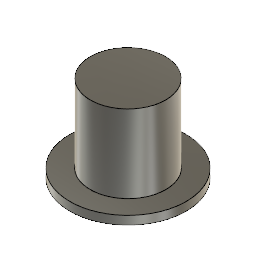
RetroconsoleButtoncap (Autodesk Fusion 360 design; units mm, degrees)
Autodesk Fusion 360 part; units mm, degrees
sketch "Sketch1" plane through (0, 0, 0) normal (0, 0, 1) x (1, 0, 0)
  circle A0 centre (0, 0) radius 4.375
  circle A1 centre (0, 0) radius 6.75
  dimension "d1" = 8.75
  dimension "d2" = 13.5
  constraint coincident A0.centre A1.centre
  measures "d1" diameter of A0
  measures "d2" diameter of A1
extrude "Extrude2" add sketch "Sketch1" along normal blind 7 contours A0 makes body 1
extrude "Extrude1" add sketch "Sketch1" along normal blind 1.5 separate body makes body 2
sketch "Sketch2" plane through (0, 0, 0) normal (0, 0, 1) x (1, 0, 0)
  circle A0 centre (0, 0) radius 3.525
  dimension "d7" = 7.05
  constraint coincident A0.centre origin
  measures "d7" diameter of A0
extrude "Extrude3" add 1 faces at (5.9169, -0.5527, 1.5) along direction (0, 0, 1) blind 0.5 on bodies 2 bodies 2 1
extrude "Extrude4" cut sketch "Sketch2" along normal blind 2 bodies 2
move_body "Move1" bodies 2 to x (1, 0, 0) y (0, -1, 0) z (0, 0, -1) at (0, 0, 0)
move_body "Move2" bodies 2 to x (1, 0, 0) y (0, -1, 0) z (0, 0, -1) at (0, -12, -14)
extrude "Extrude5" cut 1 faces at (5.9169, -12.5527, -12) along direction (0, 0, -1) blind 1 on bodies 2 bodies 2
extrude "Extrude6" add 1 faces at (-1.6096, -11.0197, -7) along direction (0, 0, 1) blind 3 on bodies 2 bodies 2
extrude "Extrude7" add 1 faces at (5.9169, -12.5527, -13) along direction (0, 0, 1) blind 0.5 on bodies 2 bodies 2
extrude "Extrude8" cut 1 faces at (5.9169, -12.5527, -12.5) along direction (0, 0, -1) blind 0.5 on bodies 2 bodies 2
